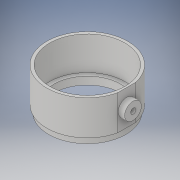
# Autodesk Inventor part: microscope_holder
Saved by Autodesk Inventor 2019 (Build 230136000, 136)
## iProperties
Created: 2019-01-11
Part Number: microscope_holder
Material: Generic
Document SubType Name: Modeling
Designer: bassp
Density: 1 g/cm^3
Appearance: Default
Author: bassp
Autodesk Inventor part; units mm, degrees
ref_plane "YZ Plane" through (0, 0, 0) normal (1, 0, 0) x (0, 1, 0)
ref_plane "XZ Plane" through (0, 0, 0) normal (0, 1, 0) x (-1, 0, 0)
ref_plane "XY Plane" through (0, 0, 0) normal (0, 0, 1) x (1, 0, 0)
sketch "Sketch1" plane through (0, 0, 0) normal (0, 0, 1) x (1, 0, 0)
  point P0 (0, 0)
sketch "Sketch2" plane through (0, 0, 0) normal (0, 1, 0) x (-1, 0, 0)
  arc A0 (-30.6952, -7.0747) -> (-30.6952, 7.0747) centre (0, 0) ccw
  line L0 (-30.6952, 7.0747) -> (-30.6952, -7.0747)
  dimension "d0" = 63
  constraints: 2 end point, 2 point on circle, 1 centre point, 1 coincident, 1 vertical
  measures "d0" diameter of A0
extrude "Extrusion1" add sketch "Sketch2" along normal blind 27
sketch "Sketch3" plane through (0, 27, 0) normal (0, 1, 0) x (0, 0, 1)
  point P0 (0, 0)
  point P1 (0, 0)
  constraints: 1 coincident
hole "Hole1" at (0, 27, 0) direction (0, -1, 0) diameter 58.5 depth 26
sketch "Sketch4" plane through (0, 0, 0) normal (0, -1, 0) x (0, 0, 1)
  circle A0 centre (0, 0) radius 30
  dimension "d11" = 60
  constraints: 1 centre point, 1 coincident
  measures "d11" diameter of A0
extrude "Extrusion2" add sketch "Sketch4" along normal blind 5
sketch "Sketch5" plane through (0, -5, 0) normal (0, -1, 0) x (1, 0, 0)
  point P0 (0, 0)
  point P1 (0, 0)
  constraints: 1 coincident
hole "Hole2" at (0, -5, 0) direction (0, 1, 0) diameter 51.8 depth 11
sketch "Sketch6" plane through (30.6952, 0, 7.0747) normal (1, 0, 0) x (0, 0, -1)
  circle A0 centre (6.9063, 13.867) radius 6.5
  point P0 (7.0747, 0)
  dimension "d23" = 13
  constraints: 1 centre point
  measures "d23" diameter of A0
extrude "Extrusion3" add sketch "Sketch6" along normal blind 5
sketch "Sketch7" plane through (35.6952, 13.867, 0.1684) normal (1, 0, 0) x (0, 0, -1)
  point P0 (0.1684, -13.867)
  point P1 (0.2284, -0.2272)
hole "Hole3" at (35.6952, 13.6397, -0.06) direction (-1, 0, 0) diameter 4.1 depth 10
body "Solid1"
